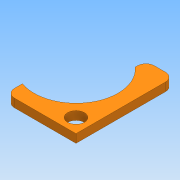
# Autodesk Inventor part: Pancake_Reverse Lever
Saved by Autodesk Inventor 2018.1 (Build 221171000, 171)
## iProperties
Created: 2019-02-27
Part Number: Pancake_Reverse Lever
Material: Nylon 6/6
Document SubType Name: Modeling
Designer: James
Density: 1.13 g/cm^3
Appearance: Orange
Mass: 1.37742 g
Surface Area: 12.4602 cm^2
Volume: 1.21896 cm^3
Author: James
Autodesk Inventor part; units mm, degrees
ref_plane "YZ Plane" through (0, 0, 0) normal (1, 0, 0) x (0, 1, 0)
ref_plane "XZ Plane" through (0, 0, 0) normal (0, 1, 0) x (-1, 0, 0)
ref_plane "XY Plane" through (0, 0, 0) normal (0, 0, 1) x (1, 0, 0)
sketch "Sketch1" plane through (0, 0, 0) normal (0, 0, 1) x (1, 0, 0)
  circle A0 centre (0, 0) radius 3
  line L0 (5, -5) -> (-20, -5)
  line L1 (-20, -5) -> (-20, 30)
  line L2 (-20, 30) -> (5, 30)
  line L3 (5, 30) -> (5, -5)
  circle A1 centre (-15, 15) radius 15
  line L4 (-20, 30) -> (-5, 30)
  line L5 (-5, 30) -> (-5, 25)
  line L6 (-5, 25) -> (-20, 25)
  line L7 (-20, 25) -> (-20, 30)
  dimension "d0" = 6
  dimension "d1" = 5
  dimension "d2" = 5
  dimension "d5" = 30
  dimension "d6" = 15
  dimension "d7" = 15
  dimension "d8" = 35
  dimension "d9" = 15
  dimension "d15" = 25
  dimension "d16" = 5
  constraints: 16 end point, 4 parallel, 2 centre point, 2 coincident, 2 horizontal, 2 perpendicular, 1 point on line, 1 tangent
  measures "d0" diameter of A0
  measures "d1" distance from line of L0 point (0, 0)
  measures "d2" distance from line of L3 point (0, 0)
  measures "d5" diameter of A1
  measures "d6" horizontal distance of point (0, 0) A1.centre
  measures "d7" horizontal distance of point (0, 0) A1.centre
  measures "d8" distance of L2.end L0.start
  measures "d9" distance of L5.end L6.end
  measures "d15" distance of L0.start L0.end
  measures "d16" distance of L4.end L5.end
extrude "Extrusion1" add sketch "Sketch1" along normal blind 3 contours L0 L1 A1 L5 L2 L3
fillet "Fillet1" radius 3 3 edges at (-5, 30, 1.5) (5, 30, 1.5) (-20, -5, 1.5)
equation "\"d7\" = d6"
body "Solid1"
